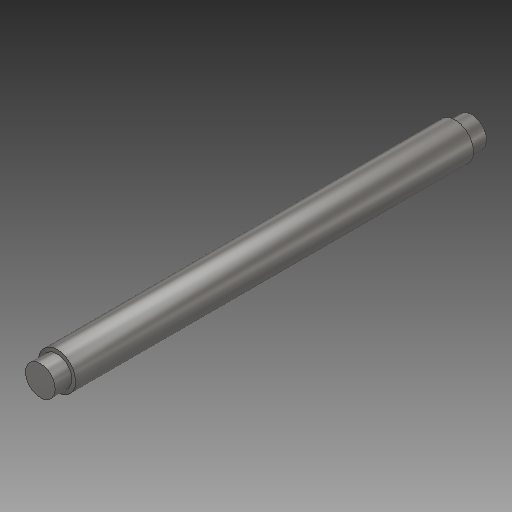
# Autodesk Inventor part: Module Pneumatic Axle
Saved by Autodesk Inventor 2019.4 (Build 234330000, 330)
## iProperties
Created: 2019-10-19
Part Number: Module Pneumatic Axle
Material: Stainless Steel
Document SubType Name: Modeling
Designer: admin
Density: 8 g/cm^3
Appearance: Semi-Polished
Author: admin
Autodesk Inventor part; units mm, degrees
ref_plane "YZ Plane" through (0, 0, 0) normal (1, 0, 0) x (0, 1, 0)
ref_plane "XZ Plane" through (0, 0, 0) normal (0, 1, 0) x (-1, 0, 0)
ref_plane "XY Plane" through (0, 0, 0) normal (0, 0, 1) x (1, 0, 0)
sketch "Sketch1" plane through (0, 0, 0) normal (1, 0, 0) x (0, 1, 0)
  line L0 (0, 0) -> (4, 0)
  line L1 (4, 0) -> (4, -4.5)
  line L2 (4, -4.5) -> (5, -4.5)
  line L3 (5, -4.5) -> (5, -111.5)
  line L4 (5, -111.5) -> (4, -111.5)
  line L5 (4, -111.5) -> (4, -116)
  line L6 (4, -116) -> (0, -116)
  line L7 (0, -116) -> (0, 0)
  dimension "d0" = 4.5
  dimension "d1" = 4.5
  dimension "d2" = 5
  dimension "d3" = 4
  dimension "d4" = 116
  constraints: 16 end point, 6 perpendicular, 2 point on line, 1 horizontal
  measures "d0" distance of L0.end L1.end
  measures "d1" distance of L4.end L5.end
  measures "d2" distance between parallel lines of L7 L3
  measures "d3" distance between parallel lines of L7 L1
  measures "d4" distance of L6.end L0.start
revolve "Revolution1" add sketch "Sketch1" angle 360 about axis through (0, 0, -116) along (0, 0, 1)
body "Solid1"
